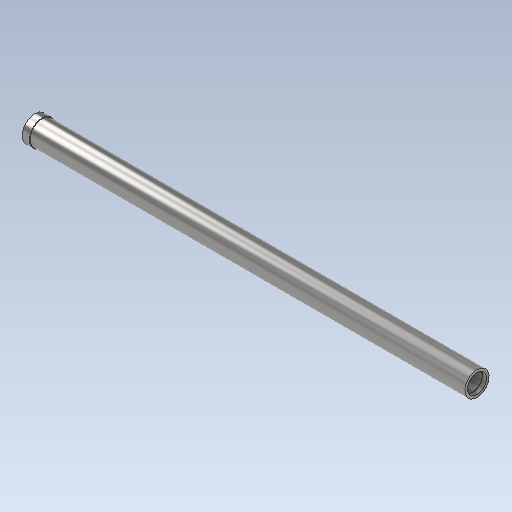
# Autodesk Inventor part: Lift.02.00.00.02
Saved by Autodesk Inventor 2021 (Build 250183000, 183)
## iProperties
Created: 2020-09-20
Part Number: Lift.02.00.00.02
Material: Сталь нержавеющая, 440C
Document SubType Name: Modeling
Designer: Kostya
Density: 7.75 g/cm^3
Appearance: С умеренной полировкой
Author: Kostya
Autodesk Inventor part; units mm, degrees
ref_plane "YZ Plane" through (0, 0, 0) normal (1, 0, 0) x (0, 1, 0)
ref_plane "XZ Plane" through (0, 0, 0) normal (0, 1, 0) x (-1, 0, 0)
ref_plane "XY Plane" through (0, 0, 0) normal (0, 0, 1) x (1, 0, 0)
sketch "Эскиз1" plane through (0, 0, 0) normal (0, 0, 1) x (1, 0, 0)
  line L0 (0, 0) -> (-3944.82, 0)
  line L1 (0, 0) -> (0, 85)
  line L2 (0, 85) -> (-3050, 85)
  line L3 (-3050, 85) -> (-3050, 90)
  line L4 (-3050, 90) -> (-3100, 90)
  line L5 (-3100, 90) -> (-3100, 0)
  line L6 (0, 67.5) -> (-30, 67.5)
  line L7 (-30, 67.5) -> (-30, 70)
  line L8 (-30, 70) -> (-3100, 70)
  dimension "d0" = 135
  dimension "d1" = 30
  dimension "d2" = 140
  dimension "d4" = 50
  dimension "d5" = 180
  dimension "d6" = 170
  dimension "d7" = 3100
  constraints: 18 end point, 6 perpendicular, 3 point on line, 2 horizontal, 1 vertical
  measures "d0" diameter of L6 L0
  measures "d1" distance of L6.start L6.end
  measures "d2" diameter of L8 L0
  measures "d4" distance of L3.end L4.end
  measures "d5" diameter of L4 L0
  measures "d6" diameter of L2 L0
  measures "d7" distance between parallel lines of L1 L5
revolve "Вращение1" add sketch "Эскиз1" angle 360 about axis through (0, 0, 0) along (-1, 0, 0) contours L6 L7 L8 L5 L4 L3 L2 L1
